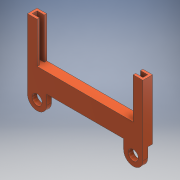
# Autodesk Inventor part: Electronics-Wedge-small
Saved by Autodesk Inventor 2018 (Build 220112000, 112)
## iProperties
Created: 2018-07-29
Part Number: Electronics-Wedge-small
Material: Generic
Document SubType Name: Modeling
Designer: jklei
Density: 1 g/cm^3
Appearance: Default
Author: jklei
Autodesk Inventor part; units mm, degrees
ref_plane "YZ Plane" through (0, 0, 0) normal (1, 0, 0) x (0, 1, 0)
ref_plane "XZ Plane" through (0, 0, 0) normal (0, 1, 0) x (-1, 0, 0)
sketch "Sketch1" plane through (0, 0, 0) normal (0, 1, 0) x (-1, 0, 0)
  line L0 (-2, -25) -> (-50, -25)
  line L1 (-50, -25) -> (-50, 0)
  line L2 (-2, 0) -> (-2, -25)
  line L3 (0, 0) -> (-2, 0)
  line L4 (-46, 0) -> (-50, 0)
  line L5 (-6, -17) -> (-46, -17)
  line L6 (-46, -17) -> (-46, 0)
  line L7 (-6, 0) -> (-6, -17)
  line L8 (-2, 0) -> (-6, 0)
  line L9 (-50, 0) -> (-46, 0)
  line L10 (-2, 0) -> (0, 0)
  dimension "d3" = 48
  dimension "d4" = 40
  dimension "d7" = 4
  dimension "d8" = 4
  dimension "d10" = 25
  dimension "d12" = 17
  constraints: 22 end point, 2 horizontal, 2 parallel, 2 point on line, 1 perpendicular
  measures "d3" distance of L0.start L0.end
  measures "d4" distance of L5.start L5.end
  measures "d7" distance between parallel lines of L2 L7
  measures "d8" distance between parallel lines of L1 L6
  measures "d10" distance of L0.end L1.end
  measures "d12" distance of L5.end L6.end
extrude "Extrusion1" add sketch "Sketch1" along normal blind 4
sketch "Sketch2" plane through (0, 0, 0) normal (0, -1, 0) x (1, 0, 0)
  circle A0 centre (6, -29) radius 2.1
  arc A1 (2, -29) -> (10, -29) centre (6, -29) ccw
  line L0 (50, -25) -> (2, -25) projected
  line L1 (2, -25) -> (2, 0) projected
  line L2 (2, -25) -> (2, -29)
  line L3 (10, -29) -> (10, -25)
  circle A2 centre (46, -29) radius 2.1
  arc A3 (42, -29) -> (50, -29) centre (46, -29) ccw
  line L4 (50, 0) -> (50, -25) projected
  line L5 (50, -25) -> (50, -29)
  line L6 (42, -29) -> (42, -25)
  point P0 (0, 0)
  dimension "d13" = 4.2
  dimension "d14" = 8
  dimension "d15" = 4
  dimension "d16" = 4
  dimension "d17" = 4.2
  dimension "d18" = 8
  dimension "d19" = 4
  dimension "d20" = 4
  constraints: 8 end point, 4 centre point, 4 point on circle, 2 coincident, 2 point on line, 2 vertical, 1 parallel, 1 perpendicular
  measures "d13" diameter of A0
  measures "d14" diameter of A1
  measures "d15" distance from line of L0 A0.centre
  measures "d16" distance from line of L1 A0.centre
  measures "d17" diameter of A2
  measures "d18" diameter of A3
  measures "d19" distance from line of L0 A2.centre
  measures "d20" distance from line of L4 A2.centre
extrude "Extrusion2" add sketch "Sketch2" against normal blind 2
ref_plane "Work Plane1" through (2, 0, 0) normal (0, 0, 1) x (1, 0, 0)
sketch "Sketch3" plane through (2, 0, 0) normal (0, 0, 1) x (1, 0, 0)
  line L0 (0, 0) -> (4, 0) projected
  line L1 (4, 0) -> (4, 4) projected
  line L2 (0, 4) -> (4, 4) projected
  line L3 (0, 0) -> (0, 4) projected
  line L4 (44, 0) -> (48, 0) projected
  line L5 (48, 0) -> (48, 4) projected
  line L6 (44, 4) -> (48, 4) projected
  line L7 (44, 0) -> (44, 4) projected
  line L8 (1, 3) -> (4, 3)
  line L9 (4, 3) -> (4, 1)
  line L10 (4, 1) -> (1, 1)
  line L11 (1, 1) -> (1, 3)
  line L12 (44, 3) -> (47, 3)
  line L13 (47, 3) -> (47, 1)
  line L14 (47, 1) -> (44, 1)
  line L15 (44, 1) -> (44, 3)
  point P0 (-2, 0)
  dimension "d24" = 3
  dimension "d25" = 2
  dimension "d26" = 1
  dimension "d27" = 0
  dimension "d28" = 3
  dimension "d29" = 2
  dimension "d30" = 1
  dimension "d31" = 0
  constraints: 16 end point, 4 parallel, 2 horizontal, 2 perpendicular
  measures "d24" distance of L9.end L10.end
  measures "d25" distance of L8.end L9.end
  measures "d26" distance between parallel lines of L0 L10
  measures "d27" distance between parallel lines of L1 L9
  measures "d28" distance of L13.end L14.end
  measures "d29" distance of L12.end L13.end
  measures "d30" distance between parallel lines of L4 L14
  measures "d31" distance between parallel lines of L7 L15
extrude "Extrusion3" cut sketch "Sketch3" against normal up to surface (17 mm away) contours L10 L11 L8 L1 | L7 L12 L13 L14
body "Solid1"
